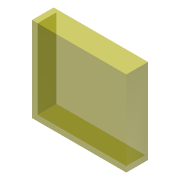
# Autodesk Inventor part: Vat
Saved by Autodesk Inventor 2014 (Build 180170000, 170)
## iProperties
Created: 2014-08-10
Part Number: Vat
Material: Generic
Document SubType Name: Modeling
Designer: Peele
Density: 1 g/cm^3
Appearance: Clear - Yellow
Author: Peele
Autodesk Inventor part; units mm, degrees
ref_plane "YZ Plane" through (0, 0, 0) normal (1, 0, 0) x (0, 1, 0)
ref_plane "XZ Plane" through (0, 0, 0) normal (0, 1, 0) x (-1, 0, 0)
ref_plane "XY Plane" through (0, 0, 0) normal (0, 0, 1) x (1, 0, 0)
sketch "Sketch1" plane through (0, 0, 0) normal (0, 1, 0) x (-1, 0, 0)
  line L0 (-50, -45) -> (50, -45)
  line L1 (50, -45) -> (50, 45)
  line L2 (50, 45) -> (-50, 45)
  line L3 (-50, 45) -> (-50, -45)
  line L4 (-50, -45) -> (50, 45) construction
  line L5 (50, -45) -> (-50, 45) construction
  point P0 (0, 0)
  dimension "d0" = 100
  dimension "d1" = 90
  constraints: 12 end point, 2 midpoint, 2 parallel, 1 horizontal, 1 perpendicular
  measures "d0" distance of L1.end L2.end
  measures "d1" distance of L0.end L1.end
extrude "Extrusion1" add sketch "Sketch1" along normal blind 3
sketch "Sketch2" plane through (0, 3, 0) normal (0, 1, 0) x (1, 0, 0)
  line L0 (50, 45) -> (-50, 45) projected
  line L1 (-50, 45) -> (-50, -45) projected
  line L2 (-50, -45) -> (50, -45)
  line L3 (50, -45) -> (50, 45)
  line L4 (50, 45) -> (-50, 45)
  line L5 (-50, 45) -> (-50, -45)
  line L6 (-50, -45) -> (50, 45) construction
  line L7 (50, -45) -> (-50, 45) construction
  line L8 (-47, -42) -> (47, -42)
  line L9 (47, -42) -> (47, 42)
  line L10 (47, 42) -> (-47, 42)
  line L11 (-47, 42) -> (-47, -42)
  line L12 (-47, -42) -> (47, 42) construction
  line L13 (47, -42) -> (-47, 42) construction
  point P0 (0, 0)
  point P1 (0, 0)
  dimension "d4" = 3
  dimension "d5" = 3
  constraints: 24 end point, 4 midpoint, 4 parallel, 2 horizontal, 2 perpendicular
  measures "d4" distance between parallel lines of L0 L10
  measures "d5" distance between parallel lines of L1 L11
extrude "Extrusion2" add sketch "Sketch2" along normal blind 20
body "Solid1"
